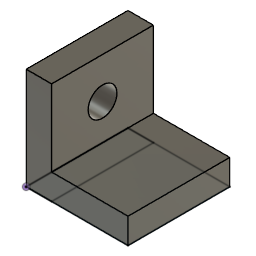
Coil housing with mounts (Autodesk Fusion 360 archive; units mm, degrees)
design "90 degree mount for coil housing"
part number: 2026-08-06-22-44-02-065
Autodesk Fusion 360 part; units mm, degrees
sketch "Sketch1" plane through (0, 0, 0) normal (0, 0, 1) x (1, 0, 0)
  line L0 (0, 0) -> (25.4, 0)
  line L1 (25.4, 0) -> (25.4, 25.4)
  line L2 (25.4, 25.4) -> (0, 25.4)
  line L3 (0, 25.4) -> (0, 0)
  line L4 (0, 25.4) -> (6.35, 25.4)
  line L5 (6.35, 25.4) -> (6.35, 0)
  line L6 (6.35, 0) -> (0, 0)
  line L7 (0, 0) -> (0, 25.4)
  dimension "d1" = 25.4
  dimension "d2" = 25.4
  dimension "d3" = 6.35
  constraint horizontal L0
  constraint vertical L1
  constraint horizontal L2
  constraint vertical L3
  constraint coincident L0.start L3.end
  constraint horizontal L4
  constraint vertical L5
  constraint horizontal L6
  constraint vertical L7
  constraint coincident L0 L5.end
  measures "d1" distance of L0.start L0.end
  measures "d2" distance of L0.start L2.end
  measures "d3" distance of L2.end L4.end
extrude "Extrude1" add sketch "Sketch1" along normal blind 6.35 contours L0 L1 L2 L5
extrude "Extrude2" add sketch "Sketch1" along normal blind 25.4 contours L0 L2 L3 L4 L5 L6 L7
sketch "Sketch2" plane through (6.35, 0, 0) normal (1, 0, 0) x (0, 1, 0)
  line L0 (0, 6.35) -> (25.4, 6.35)
  line L1 (25.4, 6.35) -> (25.4, 25.4)
  line L2 (25.4, 25.4) -> (0, 25.4)
  line L3 (0, 25.4) -> (0, 6.35)
  circle A0 centre (12.7, 15.24) radius 3.5921
extrude "Extrude3" cut sketch "Sketch2" against normal blind 38.1 contours A0

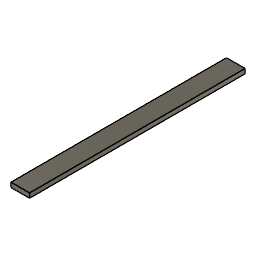
design "front and back side plates for coil housing"
part number: 2026-08-05-15-19-59-138
Autodesk Fusion 360 part; units mm, degrees
sketch "Sketch1" plane through (0, 0, 0) normal (0, 0, 1) x (1, 0, 0)
  line L0 (0, 0) -> (25.4, 0)
  line L1 (25.4, 0) -> (25.4, 293.37)
  line L2 (25.4, 293.37) -> (0, 293.37)
  line L3 (0, 293.37) -> (0, 0)
  dimension "d1" = 25.4
  dimension "d2" = 293.37
  constraint horizontal L0
  constraint vertical L1
  constraint horizontal L2
  constraint vertical L3
  constraint coincident L0.start L3.end
  measures "d1" distance of L0.start L0.end
  measures "d2" distance of L0.start L2.end
extrude "Extrude1" add sketch "Sketch1" along normal blind 6.35

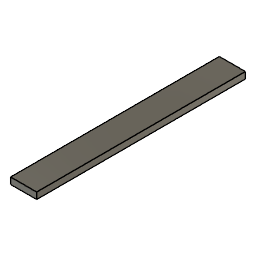
design "coil housing side plates"
part number: 2026-08-05-15-19-17-002
Autodesk Fusion 360 part; units mm, degrees
sketch "Sketch1" plane through (0, 0, 0) normal (0, 0, 1) x (1, 0, 0)
  line L0 (0, 0) -> (25.4, 0)
  line L1 (25.4, 0) -> (25.4, 203.2)
  line L2 (25.4, 203.2) -> (0, 203.2)
  line L3 (0, 203.2) -> (0, 0)
  dimension "d1" = 25.4
  dimension "d2" = 203.2
  constraint horizontal L0
  constraint vertical L1
  constraint horizontal L2
  constraint vertical L3
  constraint coincident L0.start L3.end
  measures "d1" distance of L0.start L0.end
  measures "d2" distance of L0.start L2.end
extrude "Extrude1" add sketch "Sketch1" along normal blind 6.35

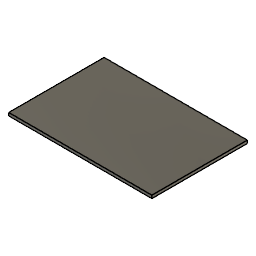
design "coil housing bottom and top plate"
part number: 2026-08-05-15-10-08-862
Autodesk Fusion 360 part; units mm, degrees
sketch "Sketch1" plane through (0, 0, 0) normal (0, 0, 1) x (1, 0, 0)
  line L0 (152.4, 101.6) -> (-152.4, 101.6)
  line L1 (-152.4, 101.6) -> (-152.4, -101.6)
  line L2 (-152.4, -101.6) -> (152.4, -101.6)
  line L3 (152.4, -101.6) -> (152.4, 101.6)
  line L4 (152.4, 101.6) -> (-152.4, -101.6) construction
  line L5 (-152.4, 101.6) -> (152.4, -101.6) construction
  dimension "d1" = 304.8
  dimension "d2" = 203.2
  constraint horizontal L0
  constraint perpendicular L0 L1
  constraint parallel L0 L2
  constraint parallel L1 L3
  constraint coincident L4 origin
  constraint coincident L5 origin
  measures "d1" distance of L1.end L2.end
  measures "d2" distance of L0.end L1.end
extrude "Extrude1" add sketch "Sketch1" along normal blind 6.35
